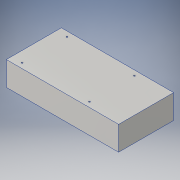
# Autodesk Inventor part: Power_Supply_S_90_18
Saved by Autodesk Inventor 2016 (Build 200138000, 138)
## iProperties
Created: 2018-05-16
Part Number: Power_Supply_S_90_18
Material: Aluminum 6061
Document SubType Name: Modeling
Designer: Phil Erle
Density: 2.7 g/cm^3
Appearance: Aluminum - Flat
Author: Phil Erle
Autodesk Inventor part; units mm, degrees
ref_plane "YZ Plane" through (0, 0, 0) normal (1, 0, 0) x (0, 1, 0)
ref_plane "XZ Plane" through (0, 0, 0) normal (0, 1, 0) x (-1, 0, 0)
ref_plane "XY Plane" through (0, 0, 0) normal (0, 0, 1) x (1, 0, 0)
sketch "Sketch1" plane through (0, 0, 0) normal (0, 0, 1) x (1, 0, 0)
  line L0 (-100, -49) -> (100, -49)
  line L1 (100, -49) -> (100, 49)
  line L2 (100, 49) -> (-100, 49)
  line L3 (-100, 49) -> (-100, -49)
  line L4 (-100, -49) -> (100, 49) construction
  line L5 (100, -49) -> (-100, 49) construction
  point P0 (0, 0)
  dimension "d0" = 200
  dimension "d1" = 98
  constraints: 12 end point, 2 midpoint, 2 parallel, 1 horizontal, 1 perpendicular
  measures "d0" distance of L2.end L1.end
  measures "d1" distance of L1.end L0.end
extrude "Extrusion1" add sketch "Sketch1" along normal blind 43
sketch "Sketch2" plane through (0, 0, 43) normal (0, 0, 1) x (1, 0, 0)
  line L0 (-81, 40) -> (39, 40) construction
  line L1 (39, 40) -> (39, -40) construction
  line L2 (39, -40) -> (-81, -40) construction
  line L3 (-81, -40) -> (-81, 40) construction
  line L4 (-100, 49) -> (-100, -49) projected
  point P0 (0, 0)
  point P1 (39, 0)
  dimension "d4" = 120
  dimension "d5" = 80
  dimension "d6" = 19
  constraints: 8 end point, 4 coincident, 2 parallel, 1 horizontal, 1 horizontal alignment, 1 midpoint, 1 perpendicular
  measures "d4" distance of L0.start L0.end
  measures "d5" distance of L2.end L0.start
  measures "d6" distance between parallel lines of L4 L3
hole "Hole1" at (-81, 40, 43) at (-81, -40, 43) at (39, 40, 43) at (39, -40, 43) direction (0, 0, -1) diameter 2.459 depth 8.8 tip angle 118 thread size "M3x0.5" class "6H" standard "ISO Metric profile"
body "Solid1"
